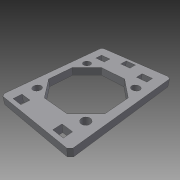
# Autodesk Inventor part: x_iddler_c_mount
Saved by Autodesk Inventor 2014 (Build 180170000, 170)
## iProperties
Created: 2013-12-02
Part Number: x_iddler_c_mount
Material: Generic
Document SubType Name: Modeling
Designer: buben
Density: 1 g/cm^3
Appearance: Default
Author: buben
Subject: Laser Cutted
Autodesk Inventor part; units mm, degrees
ref_plane "YZ Plane" through (0, 0, 0) normal (1, 0, 0) x (0, 1, 0)
ref_plane "XZ Plane" through (0, 0, 0) normal (0, 1, 0) x (-1, 0, 0)
ref_plane "XY Plane" through (0, 0, 0) normal (0, 0, 1) x (1, 0, 0)
sketch "Sketch1" plane through (0, 0, 0) normal (0, 0, 1) x (1, 0, 0)
  line L0 (0, 0) -> (60, 0)
  line L1 (60, 0) -> (60, 86)
  line L2 (60, 86) -> (0, 86)
  line L3 (0, 86) -> (0, 0)
  line L4 (54, 30.0589) -> (39.9411, 16)
  line L5 (39.9411, 16) -> (20.0589, 16)
  line L6 (20.0589, 16) -> (6, 30.0589)
  line L7 (6, 30.0589) -> (6, 49.9411)
  line L8 (6, 49.9411) -> (20.0589, 64)
  line L9 (20.0589, 64) -> (39.9411, 64)
  line L10 (39.9411, 64) -> (54, 49.9411)
  line L11 (54, 49.9411) -> (54, 30.0589)
  line L12 (9, 61) -> (51, 61) construction
  line L13 (51, 61) -> (51, 19) construction
  line L14 (51, 19) -> (9, 19) construction
  line L15 (9, 19) -> (9, 61) construction
  circle A0 centre (9, 61) radius 3.2
  circle A1 centre (9, 19) radius 3.2
  circle A2 centre (51, 19) radius 3.2
  circle A3 centre (51, 61) radius 3.2
  line L16 (8, 9) -> (16, 9)
  line L17 (16, 9) -> (16, 3)
  line L18 (16, 3) -> (8, 3)
  line L19 (8, 3) -> (8, 9)
  line L20 (44, 9) -> (52, 9)
  line L21 (52, 9) -> (52, 3)
  line L22 (52, 3) -> (44, 3)
  line L23 (44, 3) -> (44, 9)
  line L24 (8, 77) -> (16, 77)
  line L25 (16, 77) -> (16, 71)
  line L26 (16, 71) -> (8, 71)
  line L27 (8, 71) -> (8, 77)
  line L28 (44, 77) -> (52, 77)
  line L29 (52, 77) -> (52, 71)
  line L30 (52, 71) -> (44, 71)
  line L31 (44, 71) -> (44, 77)
  line L32 (26, 83) -> (34, 83)
  line L33 (34, 83) -> (34, 77)
  line L34 (34, 77) -> (26, 77)
  line L35 (26, 77) -> (26, 83)
  line L36 (12, 71) -> (12, 9) construction
  point P0 (30, 40)
  point P1 (30, 61)
  point P2 (30, 64)
  point P3 (9, 40)
  point P4 (6, 40)
  point P5 (12, 40)
  point P6 (30, 77)
  dimension "d0" = 42
  dimension "d1" = 42
  dimension "d2" = 48
  dimension "d3" = 6.4
  dimension "d4" = 6.4
  dimension "d5" = 6.4
  dimension "d6" = 6.4
  dimension "d7" = 6
  dimension "d8" = 8
  dimension "d9" = 6
  dimension "d10" = 8
  dimension "d11" = 3
  dimension "d12" = 8
  dimension "d13" = 6
  dimension "d14" = 3
  dimension "d15" = 86
  dimension "d16" = 6
  dimension "d17" = 6
  dimension "d18" = 8
  dimension "d19" = 8
  constraints: 74 end point, 14 parallel, 9 collinear, 8 midpoint, 7 horizontal, 7 perpendicular, 4 centre point, 4 coincident, 3 horizontal alignment, 2 vertical alignment, 17 other
  measures "d0" distance of L14.end L12.start
  measures "d1" distance of L12.start L12.end
  measures "d2" distance between parallel lines of L11 L7
  measures "d3" diameter of A0
  measures "d4" diameter of A3
  measures "d5" diameter of A1
  measures "d6" diameter of A2
  measures "d7" distance of L26.end L24.start
  measures "d8" distance of L24.start L24.end
  measures "d9" distance of L18.end L16.start
  measures "d10" distance of L28.start L28.end
  measures "d11" distance between parallel lines of L0 L18
  measures "d12" distance of L32.start L32.end
  measures "d13" distance of L34.end L32.start
  measures "d14" distance between parallel lines of L2 L32
  measures "d15" distance of L2.end L0.start
  measures "d16" distance between parallel lines of L3 L7
  measures "d17" distance between parallel lines of L1 L11
  measures "d18" distance between parallel lines of L3 L27
  measures "d19" distance between parallel lines of L1 L29
extrude "Extrusion1" add sketch "Sketch1" along normal blind 6
chamfer "Chamfer1" distance 2 angle 45 4 edges at (0, 0, 3) (60, 0, 3) (60, 86, 3) (0, 86, 3)
body "Solid1"
